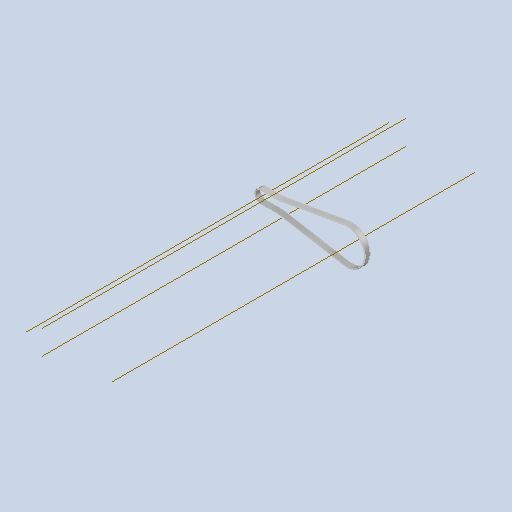
# Autodesk Inventor part: Synchronous Belt
Saved by Autodesk Inventor 2022.2 (Build 262287000, 287)
## iProperties
CustomPartVersion: 1
Created: 2022-01-08
Part Number: Synchronous Belt
Material: Rubber
Document SubType Name: Modeling
Designer: Jochen
Density: 1 g/cm^3
Appearance: Rubber - Black - Version 1.1
Author: Jochen
Autodesk Inventor part; units mm, degrees
sketch "Sketch Path" plane through (0, 0, 0) normal (0, 0, 1) x (1, 0, 0)
  arc A0 (1.9319, 18.3368) -> (1.9319, 8.7876) centre (1.9231, 13.5622) ccw
  arc A1 (16.2894, 8.7353) -> (15.407, 8.8122) centre (15.4161, 3.8122) ccw
  arc A2 (68.5875, -0.5416) -> (68.5875, 27.666) centre (71.0893, 13.5622) ccw
  arc A3 (15.407, 18.3122) -> (16.2894, 18.3891) centre (15.4161, 23.3122) ccw
  line L0 (15.407, 18.3122) -> (1.9319, 18.3368)
  line L1 (1.9319, 8.7876) -> (15.407, 8.8122)
  line L2 (16.2894, 8.7353) -> (68.5875, -0.5416)
  line L3 (68.5875, 27.666) -> (16.2894, 18.3891)
  constraints: 8 end point, 8 point on circle, 4 centre point
ref_plane "Cross Section Plane" through (1.9319, 18.3368, 0) normal (1, -0.0018, 0) x (0, 0, 1)
ref_plane "Work Plane2" through (1.9231, 13.5622, 0) normal (-1, 0, 0) x (0, 0, 1)
ref_plane "Work Plane3" through (71.0893, 13.5622, 0) normal (0.9951, -0.0987, 0) x (0, 0, 1)
sketch "Cross Section" plane through (1.9319, 18.3368, 0) normal (1, -0.0018, 0) x (0, 0, 1)
  line L0 (-2, 0.3) -> (2, 0.3)
  line L1 (2, 0.3) -> (2, -0.3)
  line L2 (2, -0.3) -> (-2, -0.3)
  line L3 (-2, -0.3) -> (-2, 0.3)
  line L4 (-2, 0) -> (2, 0) construction
  point P0 (0, 0)
  point P1 (0, 0)
  dimension "d0" = 4
  dimension "d4" = 0.3
  dimension "d5" = 0.3
  constraints: 10 end point, 3 midpoint, 2 parallel, 1 coincident, 1 horizontal, 1 perpendicular, 1 other
  measures "d0" distance between parallel lines of L1 L3
  measures "d4" distance between parallel lines of L2 L4
  measures "d5" distance between parallel lines of L4 L0
sweep "Belt" add profiles "Cross Section" path "Sketch Path"
equation "\"d0\" = da_B"
equation "\"d4\" = da_a"
equation "\"d5\" = da_a2"
equation "\"da_B\" = 4"
equation "\"da_pb\" = 2.5"
equation "\"da_a\" = 0.3"
equation "\"da_S\" = 1.5"
equation "\"da_Beta\" = 20deg"
equation "\"da_Ht\" = 0.7"
equation "\"da_H\" = 1.3"
equation "\"da_a2\" = 0.3"
body "Solid1"
